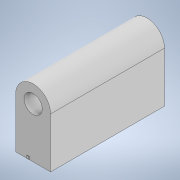
# Autodesk Inventor part: stator unit
Saved by Autodesk Inventor 2021 (Build 250183000, 183)
## iProperties
Created: 2021-04-19
Part Number: stator unit
Material: Generic
Document SubType Name: Modeling
Designer: miw14
Density: 1 g/cm^3
Appearance: Default
Author: miw14
Autodesk Inventor part; units mm, degrees
ref_plane "YZ Plane" through (0, 0, 0) normal (1, 0, 0) x (0, 1, 0)
ref_plane "XZ Plane" through (0, 0, 0) normal (0, 1, 0) x (-1, 0, 0)
ref_plane "XY Plane" through (0, 0, 0) normal (0, 0, 1) x (1, 0, 0)
sketch "Sketch1" plane through (0, 0, 0) normal (0, 0, 1) x (1, 0, 0)
  line L0 (0, 0) -> (3962.4, 0)
  line L1 (3962.4, 0) -> (3962.4, 5715)
  line L2 (3962.4, 5715) -> (0, 5715)
  line L3 (0, 5715) -> (0, 0)
  circle A0 centre (1981.2, 5715) radius 1981.2
  circle A1 centre (1981.2, 5715) radius 1034.464
  point P0 (0, 5715)
  dimension "d0" = 3962.4
  dimension "d1" = 5715
  constraints: 8 end point, 2 parallel, 1 centre point, 1 coincident, 1 horizontal, 1 midpoint, 1 perpendicular, 3 other
  measures "d0" distance of L1.end L2.end
  measures "d1" distance of L0.end L1.end
extrude "Extrusion1" add sketch "Sketch1" along normal blind 12954 contours L3 A0 L1 L0 | A0 L2 A1 | L2 A1 A0
sketch "Sketch2" plane through (0, 0, 12954) normal (0, 0, 1) x (1, 0, 0)
  line L0 (0, 0) -> (3962.4, 0) projected
  line L1 (1529.4413, 0) -> (1529.4413, 326.6177)
  line L2 (1529.4413, 326.6177) -> (1275.4413, 326.6177)
  line L3 (1275.4413, 326.6177) -> (1275.4413, 0)
  dimension "d4" = 254
  constraints: 6 end point, 2 perpendicular, 2 point on line, 1 vertical
  measures "d4" distance of L1.end L2.end
extrude "Extrusion2" add sketch "Sketch2" along normal blind 25.4
body "Solid1"
